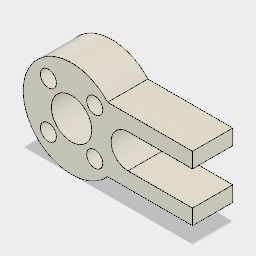
z isolator (Autodesk Fusion 360 design; units mm, degrees)
Autodesk Fusion 360 part; units mm, degrees
sketch "Sketch1" plane through (0, 0, 0) normal (0, 0, 1) x (1, 0, 0)
  circle A0 centre (0, 0) radius 12
  circle A1 centre (0, 0) radius 5
  line L0 (30, 8) -> (8.9443, 8)
  line L1 (30, 8) -> (30, 4.2)
  line L2 (30, 4.2) -> (11.241, 4.2)
  line L3 (5.75, -5.75) -> (-5.75, -5.75) construction
  line L4 (-5.75, -5.75) -> (-5.75, 5.75) construction
  line L5 (-5.75, 5.75) -> (5.75, 5.75) construction
  line L6 (5.75, 5.75) -> (5.75, -5.75) construction
  circle A2 centre (14, 0) radius 4.2
  line L7 (-5.75, 0) -> (5.75, 0) construction
  line L8 (30, -8) -> (8.9443, -8)
  line L9 (30, -8) -> (30, -4.2)
  line L10 (30, -4.2) -> (11.241, -4.2)
  dimension "d78" = 24
  dimension "d79" = 10
  dimension "d80" = 30
  dimension "d81" = 3.8
  dimension "d82" = 8
  dimension "d83" = 11.5
  dimension "d84" = 8.4
  dimension "d85" = 14
  measures "d78" diameter of A0
  measures "d79" diameter of A1
  measures "d80" distance of A0.centre L0.start
  measures "d81" distance of L0.start L1.end
  measures "d82" distance of A0.centre L0.start
  measures "d83" distance of L3.start L3.end
  measures "d84" diameter of A2
  measures "d85" distance of A0.centre A2.centre
extrude "Extrude1" add sketch "Sketch1" along normal blind 7 contours A0 A2 | A0 L2 A2 | A0 L0 L1 L2 | A0 L8 L9 L10 | A0 A2 L10 picked at (8.4877, -3.2528)
hole "Hole1" at (5.75, -5.75, 0) at (5.75, 5.75, 0) at (-5.75, 5.75, 0) at (-5.75, -5.75, 0) direction (0, 0, 1) diameter 4 end through all counterbore diameter 6 counterbore depth 4
move_face "OffsetFaces1" offset 3 1 faces at (17.6481, 6.7333, 0)
